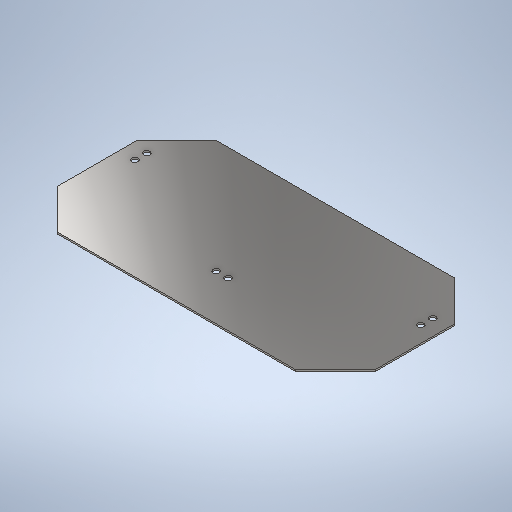
# Autodesk Inventor part: chassis up
Saved by Autodesk Inventor 2026.1 (Build 301233020, 233B)
## iProperties
Created: 2026-01-22
Part Number: chassis up
Material: Steel, Mild
Document SubType Name: Modeling
Designer: user
Density: 7.85 g/cm^3
Appearance: Semi-Polished
Mass: 3211.32 g
Surface Area: 4154.01 cm^2
Volume: 409.085 cm^3
Author: user
Autodesk Inventor part; units mm, degrees
ref_plane "YZ Plane" through (0, 0, 0) normal (1, 0, 0) x (0, 1, 0)
ref_plane "XZ Plane" through (0, 0, 0) normal (0, 1, 0) x (-1, 0, 0)
sketch "Sketch1" plane through (0, 0, 0) normal (0, 1, 0) x (-1, 0, 0)
  line L0 (-200, 300) -> (200, 300)
  line L1 (200, 300) -> (200, -300)
  line L2 (200, -300) -> (-200, -300)
  line L3 (-200, -300) -> (-200, 300)
  line L4 (-200, 300) -> (200, -300) construction
  line L5 (200, 300) -> (-200, -300) construction
  point P0 (0, 0)
  dimension "d0" = 400
  dimension "d1" = 600
  constraints: 12 end point, 2 midpoint, 2 parallel, 1 horizontal, 1 perpendicular
  measures "d0" distance of L1.end L2.end
  measures "d1" distance of L0.end L1.end
extrude "Extrusion1" add sketch "Sketch1" along normal blind 2
sketch "Sketch2" plane through (0, 2, 0) normal (0, 1, 0) x (1, 0, 0)
  line L0 (200, 300) -> (-200, 300) projected
  line L1 (-200, 300) -> (-200, 275)
  line L2 (-200, 300) -> (-200, -300) projected
  line L3 (-200, 300) -> (-100, 300)
  line L4 (-100, 300) -> (-200, 275)
  line L5 (-200, 275) -> (-200, 250)
  line L6 (-200, 250) -> (-175, 250)
  line L7 (-175, 250) -> (-175, 150)
  line L8 (-175, 150) -> (-200, 150)
  line L9 (-200, 250) -> (-200, 150)
  line L10 (0, 250) -> (0, 74.4907)
  line L11 (-155.9773, 0) -> (157.8952, 0)
  line L12 (-200, 300) -> (200, 300)
  line L13 (200, 300) -> (200, -300)
  line L14 (100, 300) -> (200, 275)
  line L15 (200, 250) -> (175, 250)
  line L16 (175, 250) -> (175, 150)
  line L17 (175, 150) -> (200, 150)
  line L18 (200, -300) -> (-200, -300)
  line L19 (-200, -300) -> (-200, -275)
  line L20 (-200, -300) -> (-100, -300)
  line L21 (-100, -300) -> (-200, -275)
  line L22 (-200, -275) -> (-200, -250)
  line L23 (-200, -250) -> (-200, -150)
  line L24 (200, -300) -> (200, 300)
  line L25 (100, -300) -> (200, -275)
  line L26 (-200, -300) -> (200, -300)
  point P0 (0, 0)
  dimension "d4" = 25
  dimension "d5" = 100
  dimension "d6" = 25
  dimension "d7" = 25
  dimension "d8" = 100
  constraints: 50 end point, 20 symmetric about line, 11 point on line, 3 perpendicular, 1 collinear, 1 horizontal, 1 vertical
  measures "d4" distance of L0.end L1.end
  measures "d5" distance of L0.end L3.end
  measures "d6" distance of L1.end L5.end
  measures "d7" distance of L5.end L6.end
  measures "d8" distance of L6.end L7.end
extrude "Extrusion2" cut sketch "Sketch2" against normal blind 2 contours L13 L14 L0 | L4 L1 L0 | L13 L17 L16 L15 | L6 L7 L8 L2 | L13 L18 L25 | L18 L2 L21
mirror "Mirror2" about plane through (0, 0, 0) normal (1, 0, 0)
ref_plane "Work Plane2" through (-100, 0, 190) normal (0, 0, 1) x (1, 0, 0)
mirror "Mirror4" about plane through (-100, 0, 190) normal (0, 0, 1) of "Mirror2"
sketch "Sketch13" plane through (0, 2, 0) normal (0, 1, 0) x (1, 0, 0)
  line L0 (-200, 150) -> (-200, -275) projected
  line L1 (-200, 0) -> (-200, 150)
  line L2 (-200, 150) -> (200, 150)
  line L3 (200, 150) -> (200, -150)
  line L4 (200, -150) -> (-200, -150)
  line L5 (-200, 0) -> (-200, 50)
  line L6 (-200, 50) -> (200, 50)
  line L7 (-200, 50) -> (-200, 595.1707)
  line L8 (-200, 595.1707) -> (291.7949, 595.1707)
  line L9 (291.7949, 595.1707) -> (291.7949, 150)
  line L10 (291.7949, 150) -> (200, 150)
  line L11 (-200, -150) -> (-200, -431.5542)
  line L12 (-200, -431.5542) -> (200, -431.5542)
  line L13 (200, -431.5542) -> (200, -150)
  point P0 (0, 0)
  dimension "d71" = 400
  dimension "d72" = 300
  dimension "d73" = 50
  constraints: 26 end point, 8 perpendicular, 6 point on line, 1 vertical
  measures "d71" distance of L0.start L2.end
  measures "d72" distance of L2.end L3.end
  measures "d73" distance of L1.start L5.end
extrude "Extrusion11" cut sketch "Sketch13" against normal blind 10 contours L2 L3 L6 L0 | L7 L8 L9 L10 L2 | L4 L13 L12 L11 L0
sketch "Sketch14" plane through (0, 2, 0) normal (0, 1, 0) x (1, 0, 0)
  line L0 (-250, 100) -> (-150, 100)
  line L1 (-150, 100) -> (-150, 0)
  line L2 (-150, 0) -> (-250, 0)
  line L3 (-250, 0) -> (-250, 100)
  line L4 (-200, 50) -> (-200, -150) projected
  line L5 (-250, 100) -> (-150, 0) construction
  line L6 (-150, 100) -> (-250, 0) construction
  line L7 (200, 50) -> (-200, 50) projected
  line L8 (-150, 50) -> (-200, 0)
  line L9 (-200, 50) -> (-200, -50)
  line L10 (-200, -50) -> (200, -50)
  line L11 (0, 0) -> (0, -87.9853)
  line L12 (-250, -200) -> (-150, -200)
  line L13 (-150, -200) -> (-150, -100)
  line L14 (-150, -100) -> (-250, -100)
  line L15 (-250, -100) -> (-250, -200)
  line L16 (-150, -150) -> (-200, -100)
  line L17 (250, 100) -> (150, 100)
  line L18 (150, 100) -> (150, 0)
  line L19 (150, 0) -> (250, 0)
  line L20 (250, 0) -> (250, 100)
  line L21 (150, 50) -> (200, 0)
  line L22 (250, -200) -> (150, -200)
  line L23 (250, -100) -> (250, -200)
  line L24 (150, -100) -> (250, -100)
  line L25 (150, -150) -> (200, -100)
  line L26 (150, -200) -> (150, -100)
  dimension "d76" = 100
  dimension "d77" = 100
  dimension "d78" = 100
  constraints: 50 end point, 18 symmetric about line, 11 midpoint, 2 parallel, 2 perpendicular, 2 point on line, 1 horizontal, 1 vertical
  measures "d76" distance of L1.end L2.end
  measures "d77" distance of L0.end L1.end
  measures "d78" distance of L4.start L9.end
extrude "Extrusion12" cut sketch "Sketch14" against normal blind 10 contours L0 L1 L7 L4 L2 L3 | L8 L4 L7 | L15 L14 L16 L13 L12 | L20 L19 L21 L18 L17 | L22 L26 L25 L24 L23
sketch "Sketch15" plane through (0, 2, 0) normal (0, 1, 0) x (1, 0, 0)
  line L0 (-200, 0) -> (-200, -100) projected
  line L1 (-200, 0) -> (-200, -30)
  line L2 (-200, -30) -> (-170, -30)
  line L3 (-170, -30) -> (-170, 0)
  line L4 (-180, -15) -> (-180, -16)
  line L5 (-180, -16) -> (-180, -15)
  line L6 (-180, -15) -> (-180, -14)
  circle A0 centre (-180, -7.5) radius 4
  circle A1 centre (-180, -22.5) radius 4
  line L7 (0, 0) -> (0, -46.3113)
  circle A2 centre (180, -7.5) radius 4
  circle A3 centre (180, -22.5) radius 4
  dimension "d81" = 30
  dimension "d82" = 30
  dimension "d86" = 1
  dimension "d89" = 8
  dimension "d99" = 15
  constraints: 14 end point, 4 centre point, 2 perpendicular, 2 point on line, 2 symmetric about line, 1 collinear, 1 vertical, 2 other
  measures "d81" distance of L0.start L1.end
  measures "d82" distance of L1.end L2.end
  measures "d86" distance of L4.start L6.end
  measures "d89" diameter of A0
  measures "d99" distance of A1.centre A0.centre
extrude "Extrusion13" cut sketch "Sketch15" against normal blind 10
sketch "Sketch16" plane through (0, 2, 0) normal (0, 1, 0) x (1, 0, 0)
  circle A0 centre (-80, -99.9978) radius 4 projected
  circle A1 centre (70, -99.9978) radius 4 projected
  circle A2 centre (7.5, -92.5769) radius 4
  circle A3 centre (-7.5, -92.5769) radius 4
  line L0 (0, -99.9978) -> (0, -89.9978)
  line L1 (0, -99.9978) -> (0, -91.9978)
  point P0 (0, 0)
  dimension "d95" = 8
  dimension "d96" = 8
  dimension "d106" = 8
  constraints: 4 end point, 2 centre point, 1 point on line, 1 vertical
  measures "d95" diameter of A2
  measures "d96" diameter of A3
  measures "d106" distance of L0.start L1.end
extrude "Extrusion14" cut sketch "Sketch16" against normal blind 10 contours A2 | A3
ref_plane "Work Plane1" through (0, 0, 0) normal (1, 0, 0) x (0, 1, 0)
ref_plane "Work Plane3" through (0, 0, 380) normal (-1, 0, 0) x (0, 1, 0)
ref_plane "Work Plane4" through (0, 0, 380) normal (-1, 0, 0) x (0, 1, 0)
body "Solid1"
